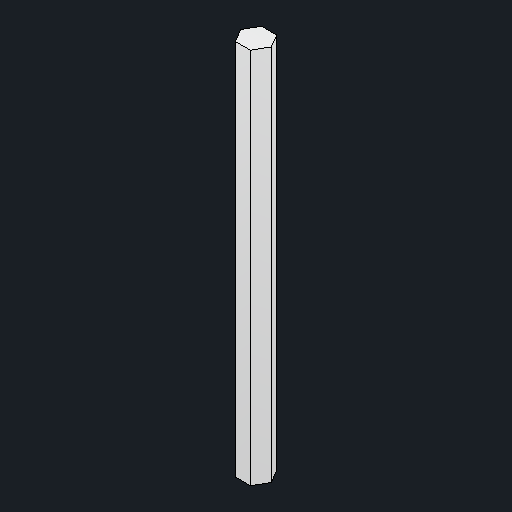
# Autodesk Inventor part: STOCK,TOP-RIGHT,HEX
Saved by Autodesk Inventor 2026.1 (Build 301233020, 233B)
## iProperties
Created: 2026-03-30
Part Number: STOCK,TOP-RIGHT,HEX
Material: Aluminum 6061
Document SubType Name: Modeling
Designer: Owen L
Density: 2.7 g/cm^3
Appearance: Aluminum - Flat
Mass: 68.8515 g
Surface Area: 83.1103 cm^2
Volume: 25.5006 cm^3
Author: Owen L
Autodesk Inventor part; units mm, degrees
ref_plane "YZ Plane" through (0, 0, 0) normal (1, 0, 0) x (0, 1, 0)
ref_plane "XZ Plane" through (0, 0, 0) normal (0, 1, 0) x (-1, 0, 0)
ref_plane "XY Plane" through (0, 0, 0) normal (0, 0, 1) x (1, 0, 0)
sketch "Sketch1" plane through (0, 0, 0) normal (0, 1, 0) x (-1, 0, 0)
  line L0 (-3.6662, -6.35) -> (-7.3323, 0)
  line L1 (-7.3323, 0) -> (-3.6662, 6.35)
  line L2 (-3.6662, 6.35) -> (3.6662, 6.35)
  line L3 (3.6662, 6.35) -> (7.3323, 0)
  line L4 (7.3323, 0) -> (3.6662, -6.35)
  line L5 (3.6662, -6.35) -> (-3.6662, -6.35)
  point P0 (0, 0)
  point P1 (0, 0)
  dimension "d0" = 12.7
  constraints: 12 end point, 1 coincident, 1 horizontal, 13 other
  measures "d0" distance between parallel lines of L2 L5
extrude "Extrusion1" add sketch "Sketch1" along normal blind 182.5625
body "Solid1"
